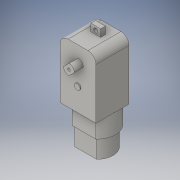
# Autodesk Inventor part: Motor
Saved by Autodesk Inventor 2016 (Build 200138000, 138)
## iProperties
Created: 2017-09-12
Part Number: Motor
Material: Generic
Document SubType Name: Modeling
Designer: student
Density: 1 g/cm^3
Appearance: Default
Author: student
Autodesk Inventor part; units mm, degrees
ref_plane "YZ Plane" through (0, 0, 0) normal (1, 0, 0) x (0, 1, 0)
ref_plane "XZ Plane" through (0, 0, 0) normal (0, 1, 0) x (-1, 0, 0)
ref_plane "XY Plane" through (0, 0, 0) normal (0, 0, 1) x (1, 0, 0)
sketch "Sketch1" plane through (0, 0, 0) normal (0, 0, 1) x (1, 0, 0)
  line L0 (-6.2484, 18.5674) -> (6.2484, 18.5674)
  line L1 (11.3284, 13.4874) -> (11.3284, -18.5674)
  line L2 (11.3284, -18.5674) -> (-11.3284, -18.5674)
  line L3 (-11.3284, -18.5674) -> (-11.3284, 13.4874)
  line L4 (-11.3284, 18.5674) -> (11.3284, -18.5674) construction
  line L5 (11.3284, 18.5674) -> (-11.3284, -18.5674) construction
  arc A0 (-6.2484, 18.5674) -> (-11.3284, 13.4874) centre (-6.2484, 13.4874) ccw
  arc A1 (11.3284, 13.4874) -> (6.2484, 18.5674) centre (6.2484, 13.4874) ccw
  point P0 (0, 0)
  dimension "d1" = 37.1348
  dimension "d2" = 5.08
  dimension "d45" = 22.6568
  constraints: 12 end point, 4 point on circle, 4 point on line, 4 tangent, 2 centre point, 2 midpoint, 2 parallel, 1 equal radius, 1 horizontal, 1 perpendicular
  measures "d1" distance of L1.end L5.start
  measures "d2" radius of A0
  measures "d45" distance of L1.end L2.end
extrude "Extrusion1" add sketch "Sketch1" along normal blind 20.828
sketch "Sketch2" plane through (0, 0, 20.828) normal (0, 0, 1) x (1, 0, 0)
  line L0 (-3.4946, 7.7761) -> (0.1481, 11.4046)
  line L1 (3.4167, 7.9922) -> (-0.097, 4.4922)
  line L2 (6.2484, 18.5674) -> (-6.2484, 18.5674) projected
  arc A0 (3.4167, 7.9922) -> (0.1481, 11.4046) centre (-0.0127, 7.9789) ccw
  arc A1 (-3.4946, 7.7761) -> (-0.097, 4.4922) centre (-0.0127, 7.9789) ccw
  point P0 (0, 0)
  dimension "d9" = 7.1628
  dimension "d11" = 4.7244
  constraints: 4 end point, 4 point on circle, 2 centre point, 1 coincident, 1 parallel
  measures "d9" distance from line of L0.end L2
  measures "d11" distance between parallel lines of L1 L0
extrude "Extrusion2" add sketch "Sketch2" along normal blind 5.6896
sketch "Sketch3" plane through (0, 0, 26.5176) normal (0, 0, 1) x (1, 0, 0)
  circle A0 centre (0, 7.9106) radius 0.8509
  point P0 (0, 0)
  dimension "d14" = 1.7018
  constraints: 1 centre point
  measures "d14" diameter of A0
extrude "Extrusion3" cut sketch "Sketch3" against normal blind 5.5372
sketch "Sketch4" plane through (-6.2484, 18.5674, 0) normal (0, 1, 0) x (1, 0, 0)
  line L0 (3.2004, -6.604) -> (9.2964, -6.604)
  line L1 (9.2964, -6.604) -> (9.2964, -9.6266)
  line L2 (9.2964, -9.6266) -> (3.2004, -9.6266)
  line L3 (3.2004, -9.6266) -> (3.2004, -6.604)
  line L4 (3.2004, -6.604) -> (9.2964, -9.6266) construction
  line L5 (9.2964, -6.604) -> (3.2004, -9.6266) construction
  line L6 (12.4968, 0) -> (0, 0) projected
  point P0 (6.2484, 0)
  point P1 (6.2484, -8.1153)
  point P2 (6.2484, -8.1153)
  point P3 (6.2484, 0)
  dimension "d17" = 6.096
  dimension "d18" = 3.0226
  dimension "d19" = 6.604
  constraints: 12 end point, 4 midpoint, 2 parallel, 1 horizontal, 1 perpendicular, 1 vertical alignment
  measures "d17" distance of L1.end L2.end
  measures "d18" distance of L1.end L0.end
  measures "d19" distance from line of L0 point (6.248, 0)
extrude "Extrusion4" add sketch "Sketch4" along normal blind 4.6736
sketch "Sketch5" plane through (-3.048, 18.5674, 9.6266) normal (0, 0, 1) x (1, 0, 0)
  circle A0 centre (3.048, 2.2411) radius 1.3462
  point P0 (3.048, -18.5674)
  dimension "d22" = 2.6924
  constraints: 1 centre point
  measures "d22" diameter of A0
extrude "Extrusion5" cut sketch "Sketch5" against normal blind 4.6736 and the other way blind 2.3368
sketch "Sketch6" plane through (0, 0, 20.828) normal (0, 0, 1) x (1, 0, 0)
  circle A0 centre (0, -4.0871) radius 1.8669
  line L0 (-0.097, 4.4922) -> (3.4167, 7.9922) projected
  point P0 (0, 0)
  dimension "d27" = 3.7338
  dimension "d28" = 6.1468
  constraints: 1 centre point, 1 vertical alignment
  measures "d27" diameter of A0
  measures "d28" distance from line of L0 A0.centre
extrude "Extrusion6" add sketch "Sketch6" along normal blind 0.508
sketch "Sketch8" plane through (-11.3284, -18.5674, 0) normal (0, -1, 0) x (1, 0, 0)
  line L0 (0, 0) -> (22.6568, 0) projected
  line L1 (3.8934, 17.0942) -> (18.7634, 17.0942)
  line L2 (22.6568, 17.0942) -> (22.6568, 0)
  line L3 (22.6568, 0) -> (0, 0)
  line L4 (0, 0) -> (0, 17.0942)
  line L5 (0, 20.828) -> (22.6568, 20.828) projected
  line L6 (22.6568, 0) -> (22.6568, 20.828) projected
  arc A0 (18.7634, 0) -> (18.7634, 17.0942) centre (11.3284, 8.5471) ccw
  arc A1 (3.8934, 17.0942) -> (3.8934, 0) centre (11.3284, 8.5471) ccw
  point P0 (11.3284, 0)
  point P1 (11.3284, 8.5471)
  point P2 (11.3284, 20.828)
  constraints: 8 end point, 4 point on circle, 3 point on line, 2 centre point, 2 parallel, 1 horizontal, 1 midpoint, 1 perpendicular, 1 tangent
extrude "Extrusion8" add sketch "Sketch8" along normal blind 12.446 contours A1 L1 A0 L0
sketch "Sketch9" plane through (-11.3284, -31.0134, 0) normal (0, -1, 0) x (1, 0, 0)
  line L0 (4.4951, 15.9258) -> (18.1617, 15.9258)
  line L1 (17.8198, 1.1684) -> (4.837, 1.1684)
  arc A0 (4.4951, 15.9258) -> (4.837, 1.1684) centre (11.3284, 8.7014) ccw
  arc A1 (17.8198, 1.1684) -> (18.1617, 15.9258) centre (11.3284, 8.7014) ccw
  line L2 (18.7634, 17.0942) -> (3.8934, 17.0942) projected
  line L3 (3.8934, 0) -> (18.7634, 0) projected
  point P0 (11.3284, 0)
  point P1 (11.3284, 8.7014)
  point P2 (11.3284, 8.7014)
  point P3 (11.3284, 8.7014)
  dimension "d53" = 1.1684
  dimension "d54" = 1.1684
  constraints: 5 coincident, 4 end point, 4 point on circle, 2 centre point, 1 horizontal, 1 parallel
  measures "d53" distance between parallel lines of L0 L2
  measures "d54" distance between parallel lines of L3 L1
extrude "Extrusion9" add sketch "Sketch9" along normal blind 11.9634
body "Solid1"
